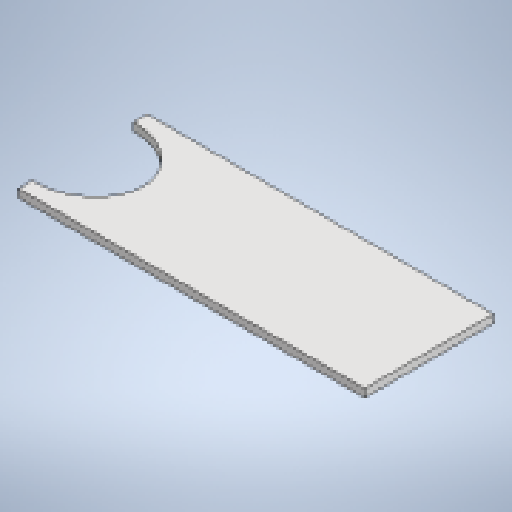
# Autodesk Inventor part: NVPH-345 feeder hose 2
Saved by Autodesk Inventor 2025.1 (Build 291241020, 241B)
## iProperties
Created: 2024-12-03
Part Number: NVPH-345 feeder hose 2
Material: Generic
Document SubType Name: Sheet Metal
Designer: admin
Density: 1 g/cm^3
Flat Pattern Width: 16 cm
Flat Pattern Length: 43 cm
Flat Pattern Area: 688 cm^2
Sheet Metal Rule: Default_mm
Sheet Metal Width: 160.000 mm
Sheet Metal Length: 430.000 mm
Sheet Metal Area: 68800.000 mm^2
Appearance: Default
Mass: 570.78 g
Surface Area: 1266.68 cm^2
Volume: 570.78 cm^3
Author: user
Autodesk Inventor part; units mm, degrees
ref_plane "YZ Plane" through (0, 0, 0) normal (1, 0, 0) x (0, 1, 0)
ref_plane "XZ Plane" through (0, 0, 0) normal (0, 1, 0) x (-1, 0, 0)
ref_plane "XY Plane" through (0, 0, 0) normal (0, 0, 1) x (1, 0, 0)
sketch "Sketch1" plane through (0, 0, 0) normal (0, 0, 1) x (1, 0, 0)
  ellipse E0 centre (0, 0) end of major axis (75, 0) minor radius 63
  line L0 (0, -63) -> (0, -80)
  line L1 (0, -80) -> (430, -80)
  line L2 (430, -80) -> (430, 80)
  line L3 (430, 80) -> (0, 80)
  line L4 (0, 80) -> (0, 63)
  line L5 (0, 0) -> (430, 0) construction
  point P0 (0, 71.5)
  dimension "d12" = 75
  dimension "d13" = 63
  dimension "d14" = 160
  dimension "d15" = 430
  measures "d14" distance between parallel lines of L3 L1
  measures "d15" distance of L2.end L3.end
extrude "Plate1" add sketch "Sketch1" along normal blind 10 contours E0 L4 L3 L2 L1 L0
equation "\"d16\" = Thickness"
equation "\"BendReliefDepth\" = 0.5 * Thickness"
equation "\"Thickness\" = 10"
body "Solid2"
